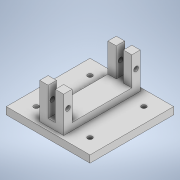
# Autodesk Inventor part: camera_plate
Saved by Autodesk Inventor 2020 (Build 240168000, 168)
## iProperties
Created: 2020-02-09
Part Number: camera_plate
Material: Generic
Document SubType Name: Modeling
Designer: mdjb501
Density: 1 g/cm^3
Appearance: Default
Author: mdjb501
Autodesk Inventor part; units mm, degrees
ref_plane "YZ Plane" through (0, 0, 0) normal (1, 0, 0) x (0, 1, 0)
ref_plane "XZ Plane" through (0, 0, 0) normal (0, 1, 0) x (-1, 0, 0)
ref_plane "XY Plane" through (0, 0, 0) normal (0, 0, 1) x (1, 0, 0)
sketch "Sketch1" plane through (0, 0, 0) normal (0, 1, 0) x (-1, 0, 0)
  circle A0 centre (11.25, 11.25) radius 1
  circle A1 centre (11.25, -11.25) radius 1
  circle A2 centre (-11.25, 11.25) radius 1
  circle A3 centre (-11.25, -11.25) radius 1
  line L0 (-17.5, 17.5) -> (17.5, 17.5)
  line L1 (17.5, 17.5) -> (17.5, -17.5)
  line L2 (17.5, -17.5) -> (-17.5, -17.5)
  line L3 (-17.5, -17.5) -> (-17.5, 17.5)
  line L4 (-5, 16) -> (5, 16)
  line L5 (5, 16) -> (5, -16)
  line L6 (5, -16) -> (-5, -16)
  line L7 (-5, -16) -> (-5, 16)
  line L8 (-5, -16) -> (-1.5, -16)
  line L9 (-1.5, -16) -> (-1.5, -12.5)
  line L10 (-1.5, -12.5) -> (-5, -12.5)
  line L11 (-5, -12.5) -> (-5, -16)
  line L12 (5, -16) -> (1.5, -16)
  line L13 (1.5, -16) -> (1.5, -12.5)
  line L14 (1.5, -12.5) -> (5, -12.5)
  line L15 (5, -12.5) -> (5, -16)
  line L16 (-5, 16) -> (-1.5, 16)
  line L17 (-1.5, 16) -> (-1.5, 12.5)
  line L18 (-1.5, 12.5) -> (-5, 12.5)
  line L19 (-5, 12.5) -> (-5, 16)
  line L20 (5, 16) -> (1.5, 16)
  line L21 (1.5, 16) -> (1.5, 12.5)
  line L22 (1.5, 12.5) -> (5, 12.5)
  line L23 (5, 12.5) -> (5, 16)
  point P0 (0, 0)
  constraints: 48 end point, 12 parallel, 6 horizontal, 6 perpendicular, 4 centre point
extrude "Extrusion1" add sketch "Sketch1" along normal blind 18 contours L4 L17 L18 L7 | L4 L5 L22 L21 | L10 L9 L6 L7 | L5 L6 L13 L14
extrude "Extrusion2" add sketch "Sketch1" along normal blind 6 contours L4 L21 L22 L5 L14 L13 L6 L9 L10 L7 L18 L17
extrude "Extrusion3" add sketch "Sketch1" along normal blind 3
sketch "Sketch2" plane through (5, 18, -12.5) normal (1, 0, 0) x (0, 0, -1)
  line L0 (-28.5, -12) -> (-25, -12) projected
  line L1 (3.5, -12) -> (0, -12) projected
  circle A0 centre (1.75, -6) radius 1
  circle A1 centre (-26.75, -6) radius 1
  point P0 (-12.5, -18)
  constraints: 2 centre point
extrude "Extrusion4" cut sketch "Sketch2" against normal blind 3.5
sketch "Sketch3" plane through (-5, 18, 12.5) normal (-1, 0, 0) x (0, 0, 1)
  circle A0 centre (-26.75, -6) radius 1 projected
  circle A1 centre (-26.75, -6) radius 1
  circle A2 centre (1.75, -6) radius 1 projected
  circle A3 centre (1.75, -6) radius 1
  point P0 (-12.5, -18)
  constraints: 2 centre point, 2 coincident
extrude "Extrusion5" cut sketch "Sketch3" against normal blind 3.5 contours A0
extrude "Extrusion6" cut sketch "Sketch3" against normal blind 3.5 contours A2
body "Solid1"
